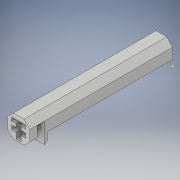
# Autodesk Inventor part: RIPnewslideholder
Saved by Autodesk Inventor 2017 (Build 210142000, 142)
## iProperties
Created: 2017-11-22
Part Number: RIPnewslideholder
Material: Generic
Document SubType Name: Modeling
Designer: build
Density: 1 g/cm^3
Appearance: Default
Author: build
Autodesk Inventor part; units mm, degrees
ref_plane "YZ Plane" through (0, 0, 0) normal (1, 0, 0) x (0, 1, 0)
ref_plane "XZ Plane" through (0, 0, 0) normal (0, 1, 0) x (-1, 0, 0)
ref_plane "XY Plane" through (0, 0, 0) normal (0, 0, 1) x (1, 0, 0)
sketch "Sketch1" plane through (0, 0, 0) normal (0, 0, 1) x (1, 0, 0)
  line L0 (0, 0) -> (0, 24.13)
  line L1 (0, 24.13) -> (24.13, 24.13)
  line L2 (24.13, 24.13) -> (24.13, 0)
  line L3 (24.13, 0) -> (0, 0)
  line L4 (0, 0) -> (0, 1.7526)
  line L5 (9.144, 1.7526) -> (14.986, 1.7526)
  line L6 (9.144, 1.7526) -> (9.271, 1.7526)
  line L7 (9.271, 1.7526) -> (14.859, 1.7526)
  line L8 (0, 0) -> (0, 7.62)
  line L9 (24.13, 0) -> (24.13, 7.62)
  line L10 (14.859, 7.62) -> (19.685, 7.62)
  line L11 (19.685, 7.62) -> (19.685, 12.319)
  line L12 (19.685, 12.319) -> (14.859, 12.319)
  line L13 (9.271, 7.62) -> (4.445, 7.62)
  line L14 (4.445, 7.62) -> (4.445, 12.319)
  line L15 (4.445, 12.319) -> (9.271, 12.319)
  line L16 (9.271, 7.62) -> (9.271, 1.7526)
  line L17 (14.859, 1.7526) -> (14.859, 7.62)
  line L18 (14.859, 12.319) -> (14.859, 15.748)
  line L19 (9.271, 12.319) -> (9.271, 15.748)
  line L20 (19.812, 15.748) -> (19.812, 19.685)
  line L21 (14.859, 15.748) -> (19.812, 15.748)
  line L22 (19.812, 19.685) -> (4.445, 19.685)
  line L23 (4.445, 19.685) -> (4.445, 15.748)
  line L24 (4.445, 15.748) -> (9.271, 15.748)
  dimension "d0" = 24.13
  dimension "d1" = 24.13
  dimension "d2" = 1.7526
  dimension "d3" = 9.144
  dimension "d5" = 0.127
  dimension "d6" = 5.588
  dimension "d7" = 7.62
  dimension "d8" = 7.62
  dimension "d9" = 4.826
  dimension "d10" = 4.699
  dimension "d11" = 4.826
  dimension "d12" = 4.699
  dimension "d13" = 5.8674
  dimension "d14" = 5.8674
  dimension "d15" = 3.429
  dimension "d16" = 3.429
  dimension "d18" = 3.937
  constraints: 50 end point, 6 perpendicular, 6 point on line, 4 horizontal, 3 parallel, 3 vertical
  measures "d0" distance of L0.start L0.end
  measures "d1" distance of L0.end L1.end
  measures "d2" distance of L0.start L4.end
  measures "d3" distance of L4.end L5.start
  measures "d5" distance of L5.start L6.end
  measures "d6" distance of L6.end L7.end
  measures "d7" distance of L0.start L8.end
  measures "d8" distance of L2.end L9.end
  measures "d9" distance of L10.start L10.end
  measures "d10" distance of L10.end L11.end
  measures "d11" distance of L13.start L13.end
  measures "d12" distance of L13.end L14.end
  measures "d13" distance of L7.end L10.start
  measures "d14" distance of L13.start L6.end
  measures "d15" distance of L12.end L18.end
  measures "d16" distance of L15.end L19.end
  measures "d18" distance of L20.start L20.end
sketch "Sketch2" plane through (0, 0, 0) normal (0, 0, 1) x (1, 0, 0)
  point P0 (0, 0)
extrude "Extrusion1" add sketch "Sketch1" along normal blind 152.4
chamfer "Chamfer1" distance 6.35 angle 45 4 edges at (0, 24.13, 76.2) (24.13, 24.13, 76.2) (24.13, 0, 76.2) (0, 0, 76.2)
sketch "Sketch3" plane through (6.35, 0, 0) normal (0, -1, 0) x (1, 0, 0)
  line L0 (17.78, 0) -> (17.78, 152.4) projected
  line L1 (17.78, 152.4) -> (17.78, 144.78)
  line L2 (17.78, 144.78) -> (-6.35, 144.78)
  line L3 (2.921, 0) -> (2.921, 152.4) projected
  line L4 (-6.35, 144.78) -> (-6.35, 137.16)
  line L5 (-6.35, 152.4) -> (-6.35, 0) projected
  line L6 (-6.35, 137.16) -> (17.78, 137.16)
  line L7 (17.78, 137.16) -> (17.78, 144.78)
  dimension "d24" = 7.62
  dimension "d25" = 7.62
  constraints: 10 end point, 3 perpendicular, 3 point on line
  measures "d24" distance of L0.end L1.end
  measures "d25" distance of L2.end L4.end
extrude "Extrusion2" cut sketch "Sketch3" against normal blind 17.399
sketch "Sketch4" plane through (6.35, 0, 0) normal (0, -1, 0) x (1, 0, 0)
  line L0 (17.78, 144.78) -> (17.78, 137.16) projected
  line L1 (17.78, 137.16) -> (-6.35, 137.16)
  line L2 (-6.35, 137.16) -> (-6.35, 133.604)
  line L3 (-6.35, 133.604) -> (17.78, 133.604)
  line L4 (17.78, 133.604) -> (17.78, 137.16)
  point P0 (-6.35, 0)
  dimension "d28" = 3.556
  constraints: 8 end point, 2 parallel, 1 horizontal, 1 perpendicular
  measures "d28" distance of L2.end L1.end
extrude "Extrusion3" add sketch "Sketch4" against normal blind 1.7526
sketch "Sketch5" plane through (0, 6.35, 137.16) normal (-0.7071, -0.7071, 0) x (-0.7071, 0.7071, 0)
  point P0 (-4.4901, 137.16)
sketch "Sketch6" plane through (6.35, 0, 0) normal (0, -1, 0) x (1, 0, 0)
  point P0 (-6.35, 0)
sketch "Sketch7" plane through (6.35, 0, 0) normal (0, -1, 0) x (1, 0, 0)
  line L0 (17.78, 137.16) -> (13.1826, 137.16) projected
  line L1 (-6.35, 137.16) -> (-6.35, 0) projected
  line L2 (17.78, 137.16) -> (-6.35, 137.16)
  line L3 (-6.35, 137.16) -> (-6.35, 133.604)
  line L4 (-6.35, 133.604) -> (17.78, 133.604)
  line L5 (17.78, 133.604) -> (17.78, 137.16)
  dimension "d31" = 3.556
  constraints: 8 end point, 2 parallel, 2 perpendicular
  measures "d31" distance of L3.end L1.start
extrude "Extrusion4" add sketch "Sketch7" along normal blind 3.81
chamfer "Chamfer2" distance 2.54 angle 45 1 edges at (12.065, -3.81, 133.604)
sketch "Sketch8" plane through (24.13, 1.7526, 137.16) normal (1, 0, 0) x (0, 0, -1)
  point P0 (137.16, -1.7526)
sketch "Sketch9" plane through (6.35, 1.7526, 0) normal (0, 1, 0) x (1, 0, 0)
  line L0 (17.78, -137.16) -> (17.78, -133.604) projected
  line L1 (13.1826, -137.16) -> (17.78, -137.16) projected
  line L2 (17.78, -137.16) -> (13.1826, -137.16)
  line L3 (13.1826, -137.16) -> (13.1826, -133.604)
  line L4 (13.1826, -133.604) -> (17.78, -133.604)
  line L5 (17.78, -133.604) -> (17.78, -137.16)
  point P0 (-6.35, 0)
  constraints: 8 end point, 3 equal length, 1 perpendicular
extrude "Extrusion5" add sketch "Sketch9" along normal blind 5.08
sketch "Sketch10" plane through (6.35, 1.7526, 0) normal (0, 1, 0) x (1, 0, 0)
  point P0 (-6.35, 0)
sketch "Sketch11" plane through (0, 1.7526, 133.604) normal (-1, 0, 0) x (0, 0, 1)
  point P0 (-133.604, -1.7526)
sketch "Sketch12" plane through (0, 1.7526, 133.604) normal (-1, 0, 0) x (0, 0, 1)
  point P0 (-133.604, -1.7526)
sketch "Sketch13" plane through (6.35, 1.7526, 0) normal (0, 1, 0) x (1, 0, 0)
  line L0 (-1.7526, -133.604) -> (-1.7526, -137.16) projected
  line L1 (-6.35, -133.604) -> (17.78, -133.604) projected
  line L2 (-1.7526, -137.16) -> (-1.7526, -133.604)
  line L3 (-1.7526, -133.604) -> (-6.35, -133.604)
  line L4 (-6.35, -133.604) -> (-6.35, -137.16)
  line L5 (-6.35, -137.16) -> (-1.7526, -137.16)
  point P0 (-6.35, 0)
  constraints: 8 end point, 2 parallel, 1 perpendicular, 1 point on line, 1 vertical
extrude "Extrusion6" add sketch "Sketch13" along normal blind 5.08
body "Solid1"
